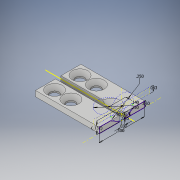
# Autodesk Inventor part: bearing_insert
Saved by Autodesk Inventor 2017 (Build 210142000, 142)
## iProperties
Created: 2017-04-27
Part Number: bearing_insert
Material: Generic
Document SubType Name: Modeling
Designer: richp
Density: 1 g/cm^3
Appearance: Default
hole1_setback: 0.280 in
hole2_setback: 0.460 in
hole_lateral: 0.140 in
bearing_thickness: 0.060 in
Author: richp
Autodesk Inventor part; units mm, degrees
ref_plane "YZ Plane" through (0, 0, 0) normal (1, 0, 0) x (0, 1, 0)
ref_plane "XZ Plane" through (0, 0, 0) normal (0, 1, 0) x (-1, 0, 0)
sketch "Sketch1" plane through (0, 0, 0) normal (1, 0, 0) x (0, 1, 0)
  line L0 (-1.3056, 0) -> (7.8339, 0) construction
  line L1 (0, -10.9768) -> (0, 10.9768) construction
  line L2 (0, -0.762) -> (0, -6.35)
  line L3 (0, -0.762) -> (0.127, -0.762)
  line L4 (0.127, -0.762) -> (1.524, -3.1817)
  line L5 (1.524, -3.1817) -> (1.524, -6.35)
  line L6 (1.524, -6.35) -> (0, -6.35)
  circle A0 centre (3.3532, 0) radius 3.175 construction
  line L7 (2.5595, 7.8406) -> (4.147, 7.8406) construction
  line L8 (4.147, 7.8406) -> (4.147, -7.8406) construction
  line L9 (4.147, -7.8406) -> (2.5595, -7.8406) construction
  line L10 (2.5595, -7.8406) -> (2.5595, 7.8406) construction
  line L11 (2.5595, 7.8406) -> (4.147, -7.8406) construction
  line L12 (4.147, 7.8406) -> (2.5595, -7.8406) construction
  line L13 (0, 0.762) -> (0, 6.35)
  line L14 (0, 0.762) -> (0.127, 0.762)
  line L15 (0.127, 0.762) -> (1.524, 3.1817)
  line L16 (1.524, 3.1817) -> (1.524, 6.35)
  line L17 (1.524, 6.35) -> (0, 6.35)
  point P0 (0, 0)
  point P1 (2.38, -3.0222)
  point P2 (2.38, 3.0222)
  dimension "d12" = 30
  dimension "d13" = 0.127
  dimension "bearing_thickness" = 1.524
  dimension "d15" = 0.762
  dimension "d17" = 6.35
  dimension "d18" = 1.5875
  dimension "d23" = 12.7
  dimension "d52" = 3.3532
  constraints: 32 end point, 5 symmetric about line, 4 perpendicular, 2 horizontal, 2 midpoint, 2 parallel, 2 point on circle, 2 point on line, 1 centre point, 1 coincident, 1 tangent
  measures "d12" angle of L1 L4
  measures "d13" distance of L2.start L3.end
  measures "bearing_thickness" distance of L5.end L2.end
  measures "d15" distance from line of point (0, 0) L3
  measures "d17" diameter of A0
  measures "d18" distance between parallel lines of L10 L8
  measures "d23" distance between parallel lines of L6 L17
  measures "d52" distance from line of L2 A0.centre
extrude "Extrusion1" add sketch "Sketch1" against normal blind 17.78
sketch "Sketch2" plane through (0, 1.524, -3.1817) normal (0, 1, 0) x (1, 0, 0)
  circle A0 centre (-3.556, -3.1817) radius 3.175 construction
  line L0 (-21.336, -3.1817) -> (3.556, -3.1817) projected
  point P0 (0, -3.1817)
  dimension "d21" = 6.35
  dimension "d22" = 3.556
  constraints: 1 centre point, 1 point on line
  measures "d21" diameter of A0
  measures "d22" distance of point (0, -3.182) A0.centre
sketch "Sketch3" plane through (-17.78, 0, 0) normal (-1, 0, 0) x (0, 0, 1)
  line L0 (0.762, 0.127) -> (0.762, 0) projected
  line L1 (0.762, 0) -> (6.35, 0) projected
  line L2 (6.35, 0) -> (6.35, 1.524) projected
  line L3 (6.35, 1.524) -> (3.1817, 1.524) projected
  line L4 (3.1817, 1.524) -> (0.762, 0.127) projected
  line L5 (0.762, 0) -> (6.35, 0) projected
  line L6 (6.35, 1.524) -> (0.762, 1.524)
  line L7 (0.762, 1.524) -> (0.762, 0)
  line L8 (0.762, 0) -> (6.35, 0)
  line L9 (6.35, 0) -> (6.35, 1.524)
  line L10 (0, -2.7581) -> (0, 4.2598) construction
  line L11 (-0.762, 0) -> (-6.35, 0)
  line L12 (-6.35, 0) -> (-6.35, 1.524)
  line L13 (-6.35, 1.524) -> (-0.762, 1.524)
  line L14 (-0.762, 1.524) -> (-0.762, 0)
  point P0 (0, 0)
  constraints: 18 end point, 4 symmetric about line, 2 parallel, 1 horizontal, 1 perpendicular, 1 point on line, 1 vertical
extrude "Extrusion2" add sketch "Sketch3" against normal blind 14.224
sketch "Sketch4" plane through (-3.556, 0, 0) normal (1, 0, 0) x (0, 0, -1)
  line L0 (-3.1817, 1.524) -> (-0.762, 0.127) projected
  line L1 (3.1817, 1.524) -> (0.762, 0.127) projected
  line L2 (-0.762, 0.127) -> (-0.762, 0) projected
  line L3 (-0.762, 0.127) -> (0.762, 0.127)
  line L4 (0, -1.3056) -> (0, 7.8339) construction
  line L5 (-0.762, 1.524) -> (-3.1817, 1.524) projected
  line L6 (-3.1817, 1.524) -> (3.1817, 1.524)
  line L7 (0, 1.524) -> (0, -0.3129)
  line L8 (-0.762, 0.127) -> (0, -0.3129)
  line L9 (0.762, 0.127) -> (0, -0.3129)
  line L10 (0.762, 0) -> (6.35, 0) projected
  point P0 (0, 0)
  point P1 (0, 0.127)
  dimension "d45" = 0.3129
  constraints: 10 end point, 3 collinear, 3 point on line, 2 midpoint, 1 perpendicular
  measures "d45" distance from line of L10 L7.end
revolve "Revolution1" [suppressed]
sketch "Sketch5" plane through (0, 1.524, -3.1817) normal (0, 1, 0) x (1, 0, 0)
  line L0 (-17.78, -2.4197) -> (-3.556, -2.4197) construction
  line L1 (-17.78, -2.4197) -> (-17.78, 3.1683) construction
  line L2 (0, 3.1683) -> (-17.78, 3.1683) construction
  line L3 (-21.336, -3.1817) -> (3.556, -3.1817) construction
  line L4 (-3.556, -3.1817) -> (-3.556, 6.3173) construction
  point P0 (0, -3.1817)
  point P1 (-10.668, 0.3743)
  point P2 (-15.24, -6.7377)
  point P3 (-10.668, -6.7377)
  point P4 (-15.24, 0.3743)
  dimension "hole1_setback" = 7.112
  dimension "hole_lateral" = 3.556
  dimension "hole2_setback" = 11.684
  constraints: 4 end point, 2 symmetric about line, 1 horizontal alignment, 1 vertical
  measures "hole1_setback" distance from line of point (-10.668, 0.374) L4
  measures "hole_lateral" distance from line of L3 point (-15.24, 0.374)
  measures "hole2_setback" distance from line of L4 point (-15.24, 0.374)
hole "Hole1" at (-10.668, 1.524, -3.556) at (-15.24, 1.524, 3.556) at (-10.668, 1.524, 3.556) at (-15.24, 1.524, -3.556) direction (0, -1, 0) diameter 2.4384 depth 25.4 tip angle 118 countersink diameter 4.3688 countersink angle 82 clearance for "Flat Head Machine Screw (82)" size "#2" standard "Ansi Unified Screw Threads"
ref_plane "Work Plane1" through (0, 3.3532, 0) normal (0, 1, 0) x (-1, 0, 0)
sketch "Sketch7" plane through (-3.556, 0, 0) normal (1, 0, 0) x (0, 0, -1)
  line L0 (3.1817, 1.524) -> (0.762, 0.127) projected
  line L1 (0.542, 0) -> (4.5015, 2.286)
  line L2 (4.5015, 2.286) -> (0.542, 0)
  line L3 (-1.1725, 2.9696) -> (0.542, 0)
  line L4 (4.5015, 2.286) -> (2.787, 5.2556)
  line L5 (2.787, 5.2556) -> (-1.1725, 2.9696)
  line L6 (10.9768, 0) -> (-10.9768, 0) construction
  point P0 (0, 0)
  dimension "d46" = 3.429
  dimension "d47" = 4.572
  constraints: 10 end point, 3 perpendicular, 2 point on line
  measures "d46" distance of L1.start L3.start
  measures "d47" distance of L4.end L3.start
revolve "Revolution3" cut sketch "Sketch7" angle 360 about axis through (-3.556, 5.2556, -2.787) along (0, -0.5, 0.8660254)
sketch "Sketch8" plane through (0, 0, 0) normal (1, 0, 0) x (0, 0, -1)
  line L0 (-0.762, 0.127) -> (-0.762, 0) projected
  line L1 (-6.35, 1.524) -> (-0.762, 1.524) projected
  line L2 (-0.762, 0) -> (-6.35, 0)
  line L3 (-6.35, 0) -> (-6.35, 1.524)
  line L4 (-6.35, 1.524) -> (-0.762, 1.524)
  line L5 (-0.762, 1.524) -> (-0.762, 0)
  line L6 (6.35, 0) -> (0.762, 0) projected
  line L7 (6.35, 1.524) -> (6.35, 0) projected
  line L8 (0.762, 0) -> (6.35, 0)
  line L9 (6.35, 0) -> (6.35, 1.524)
  line L10 (6.35, 1.524) -> (0.762, 1.524)
  line L11 (0.762, 1.524) -> (0.762, 0)
  point P0 (0, 0)
  constraints: 16 end point, 4 parallel, 2 horizontal, 2 perpendicular
extrude "Extrusion3" add sketch "Sketch8" against normal blind 3.556
sketch "Sketch9" plane through (-3.556, 0, 0) normal (-1, 0, 0) x (0, 0, 1)
  line L0 (-0.542, 0) -> (-4.5015, 2.286) projected
  line L1 (-4.5015, 2.286) -> (-2.787, 5.2556) projected
  line L2 (-2.787, 5.2556) -> (1.1725, 2.9696) projected
  line L3 (1.1725, 2.9696) -> (-0.542, 0) projected
  point P0 (0, 0)
revolve "Revolution4" cut sketch "Sketch9" angle 360 about axis through (-3.556, 5.2556, -2.787) along (0, -0.5, 0.8660254)
sketch "Sketch6" plane through (0, 3.3532, 0) normal (0, 1, 0) x (-1, 0, 0)
  circle A0 centre (3.556, 0) radius 3.175 construction
  circle A1 centre (3.556, 0) radius 3.175
  line L0 (8.0772, 0) -> (-1.3462, 0) projected
  line L1 (0.381, 0) -> (6.731, 0)
  point P0 (0, 0)
  constraints: 2 end point, 2 point on circle, 2 point on line, 1 centre point, 1 coincident, 1 concentric
revolve "Revolution2" [suppressed]
body "Solid1"
